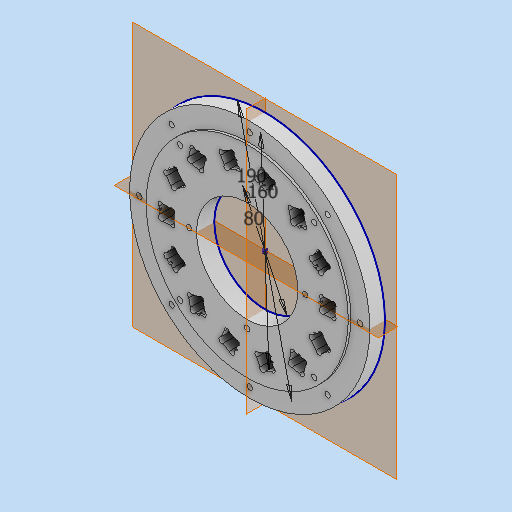
# Autodesk Inventor part: Ring 288_Final
Saved by Autodesk Inventor 2026 (Build 300175050, 175E)
## iProperties
Created: 2025-08-27
Part Number: Ring 288_Final
Material: Generic
Document SubType Name: Modeling
Designer: user
Density: 1 g/cm^3
Appearance: Default
Author: user
Autodesk Inventor part; units mm, degrees
sketch "Magnet Block n" plane through (0, 0, 0) normal (0, 0, 1) x (1, 0, 0)
  line L0 (69.7131, -5.94) -> (57.8331, -5.94)
  line L1 (57.8331, -5.94) -> (57.8331, 5.94)
  line L2 (57.8331, 5.94) -> (69.7131, 5.94)
  line L3 (69.7131, 5.94) -> (69.7131, -5.94)
  circle A0 centre (59.2461, 4.527) radius 2.1
  circle A1 centre (59.2461, -4.527) radius 2.1
  circle A2 centre (68.3001, -4.527) radius 2.1
  circle A3 centre (68.3001, 4.527) radius 2.1
  circle A4 centre (57.4731, 0) radius 0.75
  line L4 (57.4731, 0) -> (63.7731, 0)
  circle A5 centre (63.7731, 0) radius 2
  dimension "d10" = 4.2
  dimension "d11" = 4.2
  dimension "d12" = 4.2
  dimension "d13" = 4.2
  dimension "d8" = 11.88
  dimension "d9" = 11.88
  dimension "d18" = 1.5
  dimension "d19" = 6.3
  dimension "d20" = 4
  measures "d8" distance of point (57.833, 5.94) point (69.713, 5.94)
  measures "d9" distance of point (57.833, -5.94) point (57.833, 5.94)
  measures "d18" diameter of A4
  measures "d19" distance of L4.start L4.end
  measures "d20" diameter of A5
sketch "Sketch1" plane through (0, 0, 0) normal (0, 0, 1) x (1, 0, 0)
  circle A0 centre (0, 0) radius 40
  circle A1 centre (0, 0) radius 80
  circle A2 centre (0, 0) radius 95
  dimension "d0" = 80
  dimension "d1" = 160
  dimension "d2" = 190
  constraints: 3 centre point, 3 coincident
  measures "d0" diameter of A0
  measures "d1" diameter of A1
  measures "d2" diameter of A2
extrude "Extrusion1" add sketch "Sketch1" along normal blind 14 contours A1
extrude "Extrusion2" add sketch "Sketch1" along normal blind 12 contours A2
sketch "Sketch2" plane through (0, 0, 14) normal (0, 0, 1) x (1, 0, 0)
  circle A0 centre (0, 0) radius 63.7731
  line L0 (69.7131, -5.94) -> (57.8331, 5.94) construction
  line L1 (57.8331, -5.94) -> (69.7131, 5.94) construction
  line L2 (-112, 0) -> (112, 0) projected
  line L3 (69.7131, -5.94) -> (57.8331, -5.94)
  line L4 (57.8331, -5.94) -> (57.8331, 5.94)
  line L5 (57.8331, 5.94) -> (69.7131, 5.94)
  line L6 (69.7131, 5.94) -> (69.7131, -5.94)
  circle A1 centre (59.2461, 4.527) radius 2.1
  circle A2 centre (59.2461, -4.527) radius 2.1
  circle A3 centre (68.3001, -4.527) radius 2.1
  circle A4 centre (68.3001, 4.527) radius 2.1
  circle A5 centre (57.4731, 0) radius 0.75
  line L7 (57.4731, 0) -> (63.7731, 0)
  circle A6 centre (63.7731, 0) radius 2
  dimension "d7" = 127.5463
  constraints: 4 end point, 2 horizontal, 1 centre point, 1 coincident, 11 other
  measures "d7" diameter of A0
sketch "Sketch3" plane through (0, 0, 14) normal (0, 0, 1) x (1, 0, 0)
  circle A0 centre (0, 0) radius 63.7731
  line L0 (0, 0) -> (63.7731, 0)
  line L1 (0, 0) -> (57.4576, 27.6701)
  line L2 (0, 0) -> (39.7619, 49.8598)
  line L3 (0, 0) -> (14.1909, 62.1742)
  line L4 (0, 0) -> (-14.1909, 62.1742)
  line L5 (0, 0) -> (-39.7619, 49.8598)
  line L6 (0, 0) -> (-57.4576, 27.6701)
  line L7 (0, 0) -> (-63.7731, 0)
  line L8 (0, 0) -> (-57.4576, -27.6701)
  line L9 (0, 0) -> (-39.7619, -49.8598)
  line L10 (0, 0) -> (-14.1909, -62.1742)
  line L11 (0, 0) -> (14.1909, -62.1742)
  line L12 (0, 0) -> (39.7619, -49.8598)
  line L13 (0, 0) -> (57.4576, -27.6701)
  line L14 (69.7131, -5.94) -> (57.8331, -5.94)
  line L15 (57.8331, -5.94) -> (57.8331, 5.94)
  line L16 (57.8331, 5.94) -> (69.7131, 5.94)
  line L17 (69.7131, 5.94) -> (69.7131, -5.94)
  circle A1 centre (59.2461, 4.527) radius 2.1
  circle A2 centre (59.2461, -4.527) radius 2.1
  circle A3 centre (68.3001, -4.527) radius 2.1
  circle A4 centre (68.3001, 4.527) radius 2.1
  circle A5 centre (57.4731, 0) radius 0.75
  line L18 (57.4731, 0) -> (63.7731, 0)
  circle A6 centre (63.7731, 0) radius 2
  line L19 (65.8052, 28.6107) -> (58.3982, 19.3225)
  line L20 (58.3982, 19.3225) -> (49.11, 26.7296)
  line L21 (49.11, 26.7296) -> (56.5171, 36.0177)
  line L22 (56.5171, 36.0177) -> (65.8052, 28.6107)
  circle A7 centre (51.0957, 26.9533) radius 2.1
  circle A8 centre (58.1744, 21.3082) radius 2.1
  circle A9 centre (63.8195, 28.3869) radius 2.1
  circle A10 centre (56.7408, 34.032) radius 2.1
  circle A11 centre (53.5296, 22.7446) radius 0.75
  line L23 (53.5296, 22.7446) -> (57.4576, 27.6701)
  circle A12 centre (57.4576, 27.6701) radius 2
  line L24 (44.2312, 56.9727) -> (46.8747, 45.3906)
  line L25 (46.8747, 45.3906) -> (35.2926, 42.747)
  line L26 (35.2926, 42.747) -> (32.6491, 54.3291)
  line L27 (32.6491, 54.3291) -> (44.2312, 56.9727)
  circle A13 centre (36.3558, 44.439) radius 2.1
  circle A14 centre (45.1828, 46.4537) radius 2.1
  circle A15 centre (43.168, 55.2807) radius 2.1
  circle A16 centre (34.3411, 53.266) radius 2.1
  circle A17 centre (41.1638, 43.7178) radius 0.75
  line L28 (41.1638, 43.7178) -> (39.7619, 49.8598)
  circle A18 centre (39.7619, 49.8598) radius 2
  line L29 (11.4164, 70.1032) -> (22.1199, 64.9487)
  line L30 (22.1199, 64.9487) -> (16.9653, 54.2452)
  line L31 (16.9653, 54.2452) -> (6.2618, 59.3997)
  line L32 (6.2618, 59.3997) -> (11.4164, 70.1032)
  circle A19 centre (16.3054, 56.1313) radius 2.1
  circle A20 centre (20.2337, 64.2887) radius 2.1
  circle A21 centre (12.0764, 68.2171) radius 2.1
  circle A22 centre (8.148, 60.0597) radius 2.1
  circle A23 centre (19.867, 59.4407) radius 0.75
  line L33 (19.867, 59.4407) -> (14.1909, 62.1742)
  circle A24 centre (14.1909, 62.1742) radius 2
  line L34 (-22.1199, 64.9487) -> (-11.4164, 70.1032)
  line L35 (-11.4164, 70.1032) -> (-6.2618, 59.3997)
  line L36 (-6.2618, 59.3997) -> (-16.9653, 54.2452)
  line L37 (-16.9653, 54.2452) -> (-22.1199, 64.9487)
  circle A25 centre (-8.148, 60.0597) radius 2.1
  circle A26 centre (-12.0764, 68.2171) radius 2.1
  circle A27 centre (-20.2337, 64.2887) radius 2.1
  circle A28 centre (-16.3054, 56.1313) radius 2.1
  circle A29 centre (-8.5148, 64.9077) radius 0.75
  line L38 (-8.5148, 64.9077) -> (-14.1909, 62.1742)
  circle A30 centre (-14.1909, 62.1742) radius 2
  line L39 (-46.8747, 45.3906) -> (-44.2312, 56.9727)
  line L40 (-44.2312, 56.9727) -> (-32.6491, 54.3291)
  line L41 (-32.6491, 54.3291) -> (-35.2926, 42.747)
  line L42 (-35.2926, 42.747) -> (-46.8747, 45.3906)
  circle A31 centre (-34.3411, 53.266) radius 2.1
  circle A32 centre (-43.168, 55.2807) radius 2.1
  circle A33 centre (-45.1828, 46.4537) radius 2.1
  circle A34 centre (-36.3558, 44.439) radius 2.1
  circle A35 centre (-38.36, 56.0019) radius 0.75
  line L43 (-38.36, 56.0019) -> (-39.7619, 49.8598)
  circle A36 centre (-39.7619, 49.8598) radius 2
  line L44 (-58.3982, 19.3225) -> (-65.8052, 28.6107)
  line L45 (-65.8052, 28.6107) -> (-56.5171, 36.0177)
  line L46 (-56.5171, 36.0177) -> (-49.11, 26.7296)
  line L47 (-49.11, 26.7296) -> (-58.3982, 19.3225)
  circle A37 centre (-56.7408, 34.032) radius 2.1
  circle A38 centre (-63.8195, 28.3869) radius 2.1
  circle A39 centre (-58.1744, 21.3082) radius 2.1
  circle A40 centre (-51.0957, 26.9533) radius 2.1
  circle A41 centre (-61.3856, 32.5957) radius 0.75
  line L48 (-61.3856, 32.5957) -> (-57.4576, 27.6701)
  circle A42 centre (-57.4576, 27.6701) radius 2
  line L49 (-57.8331, -5.94) -> (-69.7131, -5.94)
  line L50 (-69.7131, -5.94) -> (-69.7131, 5.94)
  line L51 (-69.7131, 5.94) -> (-57.8331, 5.94)
  line L52 (-57.8331, 5.94) -> (-57.8331, -5.94)
  circle A43 centre (-68.3001, 4.527) radius 2.1
  circle A44 centre (-68.3001, -4.527) radius 2.1
  circle A45 centre (-59.2461, -4.527) radius 2.1
  circle A46 centre (-59.2461, 4.527) radius 2.1
  circle A47 centre (-70.0731, 0) radius 0.75
  line L53 (-70.0731, 0) -> (-63.7731, 0)
  circle A48 centre (-63.7731, 0) radius 2
  line L54 (-49.11, -26.7296) -> (-56.5171, -36.0177)
  line L55 (-56.5171, -36.0177) -> (-65.8052, -28.6107)
  line L56 (-65.8052, -28.6107) -> (-58.3982, -19.3225)
  line L57 (-58.3982, -19.3225) -> (-49.11, -26.7296)
  circle A49 centre (-63.8195, -28.3869) radius 2.1
  circle A50 centre (-56.7408, -34.032) radius 2.1
  circle A51 centre (-51.0957, -26.9533) radius 2.1
  circle A52 centre (-58.1744, -21.3082) radius 2.1
  circle A53 centre (-61.3856, -32.5957) radius 0.75
  line L58 (-61.3856, -32.5957) -> (-57.4576, -27.6701)
  circle A54 centre (-57.4576, -27.6701) radius 2
  line L59 (-35.2926, -42.747) -> (-32.6491, -54.3291)
  line L60 (-32.6491, -54.3291) -> (-44.2312, -56.9727)
  line L61 (-44.2312, -56.9727) -> (-46.8747, -45.3906)
  line L62 (-46.8747, -45.3906) -> (-35.2926, -42.747)
  circle A55 centre (-43.168, -55.2807) radius 2.1
  circle A56 centre (-34.3411, -53.266) radius 2.1
  circle A57 centre (-36.3558, -44.439) radius 2.1
  circle A58 centre (-45.1828, -46.4537) radius 2.1
  circle A59 centre (-38.36, -56.0019) radius 0.75
  line L63 (-38.36, -56.0019) -> (-39.7619, -49.8598)
  circle A60 centre (-39.7619, -49.8598) radius 2
  line L64 (-16.9653, -54.2452) -> (-6.2618, -59.3997)
  line L65 (-6.2618, -59.3997) -> (-11.4164, -70.1032)
  line L66 (-11.4164, -70.1032) -> (-22.1199, -64.9487)
  line L67 (-22.1199, -64.9487) -> (-16.9653, -54.2452)
  circle A61 centre (-12.0764, -68.2171) radius 2.1
  circle A62 centre (-8.148, -60.0597) radius 2.1
  circle A63 centre (-16.3054, -56.1313) radius 2.1
  circle A64 centre (-20.2337, -64.2887) radius 2.1
  circle A65 centre (-8.5148, -64.9077) radius 0.75
  line L68 (-8.5148, -64.9077) -> (-14.1909, -62.1742)
  circle A66 centre (-14.1909, -62.1742) radius 2
  line L69 (6.2618, -59.3997) -> (16.9653, -54.2452)
  line L70 (16.9653, -54.2452) -> (22.1199, -64.9487)
  line L71 (22.1199, -64.9487) -> (11.4164, -70.1032)
  line L72 (11.4164, -70.1032) -> (6.2618, -59.3997)
  circle A67 centre (20.2337, -64.2887) radius 2.1
  circle A68 centre (16.3054, -56.1313) radius 2.1
  circle A69 centre (8.148, -60.0597) radius 2.1
  circle A70 centre (12.0764, -68.2171) radius 2.1
  circle A71 centre (19.867, -59.4407) radius 0.75
  line L73 (19.867, -59.4407) -> (14.1909, -62.1742)
  circle A72 centre (14.1909, -62.1742) radius 2
  line L74 (32.6491, -54.3291) -> (35.2926, -42.747)
  line L75 (35.2926, -42.747) -> (46.8747, -45.3906)
  line L76 (46.8747, -45.3906) -> (44.2312, -56.9727)
  line L77 (44.2312, -56.9727) -> (32.6491, -54.3291)
  circle A73 centre (45.1828, -46.4537) radius 2.1
  circle A74 centre (36.3558, -44.439) radius 2.1
  circle A75 centre (34.3411, -53.266) radius 2.1
  circle A76 centre (43.168, -55.2807) radius 2.1
  circle A77 centre (41.1638, -43.7178) radius 0.75
  line L78 (41.1638, -43.7178) -> (39.7619, -49.8598)
  circle A78 centre (39.7619, -49.8598) radius 2
  line L79 (56.5171, -36.0177) -> (49.11, -26.7296)
  line L80 (49.11, -26.7296) -> (58.3982, -19.3225)
  line L81 (58.3982, -19.3225) -> (65.8052, -28.6107)
  line L82 (65.8052, -28.6107) -> (56.5171, -36.0177)
  circle A79 centre (58.1744, -21.3082) radius 2.1
  circle A80 centre (51.0957, -26.9533) radius 2.1
  circle A81 centre (56.7408, -34.032) radius 2.1
  circle A82 centre (63.8195, -28.3869) radius 2.1
  circle A83 centre (53.5296, -22.7446) radius 0.75
  line L83 (53.5296, -22.7446) -> (57.4576, -27.6701)
  circle A84 centre (57.4576, -27.6701) radius 2
  point P0 (-8.9346, 58.1126)
  point P1 (-7.549, 62.0725)
  point P2 (-10.1292, 67.4305)
  point P3 (-14.0891, 68.8161)
  point P4 (-19.4471, 66.2358)
  point P5 (-20.8328, 62.276)
  point P6 (-18.2525, 56.9179)
  point P7 (-14.2926, 55.5323)
  point P8 (-41.3391, 56.3126)
  point P9 (-44.8913, 54.0805)
  point P10 (-46.2146, 48.2827)
  point P11 (-43.9826, 44.7304)
  point P12 (-38.1848, 43.4071)
  point P13 (-34.6325, 45.6391)
  point P14 (-33.3092, 51.437)
  point P15 (-35.5412, 54.9893)
  point P16 (-54.6675, 33.6984)
  point P17 (-58.8364, 34.1681)
  point P18 (-63.4859, 30.4603)
  point P19 (-63.9556, 26.2914)
  point P20 (-60.2478, 21.6418)
  point P21 (-56.0788, 21.1721)
  point P22 (-51.4293, 24.88)
  point P23 (-50.9596, 29.0489)
  point P24 (-69.7131, -2.9735)
  point P25 (-66.7466, -5.94)
  point P26 (-60.7997, -5.94)
  point P27 (-57.8331, -2.9735)
  point P28 (-57.8331, 2.9735)
  point P29 (-60.7997, 5.94)
  point P30 (-66.7466, 5.94)
  point P31 (-69.7131, 2.9735)
  point P32 (-56.0788, -21.1721)
  point P33 (-60.2478, -21.6418)
  point P34 (-63.9556, -26.2914)
  point P35 (-63.4859, -30.4603)
  point P36 (-58.8364, -34.1681)
  point P37 (-54.6675, -33.6984)
  point P38 (-50.9596, -29.0489)
  point P39 (-51.4293, -24.88)
  point P40 (-33.3092, -51.437)
  point P41 (-34.6325, -45.6391)
  point P42 (-38.1848, -43.4071)
  point P43 (-43.9826, -44.7304)
  point P44 (-46.2146, -48.2827)
  point P45 (-44.8913, -54.0805)
  point P46 (-41.3391, -56.3126)
  point P47 (-35.5412, -54.9893)
  point P48 (-20.8328, -62.276)
  point P49 (-19.4471, -66.2358)
  point P50 (-14.0891, -68.8161)
  point P51 (-10.1292, -67.4305)
  point P52 (-7.549, -62.0725)
  point P53 (-8.9346, -58.1126)
  point P54 (-14.2926, -55.5323)
  point P55 (-18.2525, -56.9179)
  point P56 (18.2525, -56.9179)
  point P57 (14.2926, -55.5323)
  point P58 (8.9346, -58.1126)
  point P59 (7.549, -62.0725)
  point P60 (10.1292, -67.4305)
  point P61 (14.0891, -68.8161)
  point P62 (19.4471, -66.2358)
  point P63 (20.8328, -62.276)
  point P64 (38.1848, -43.4071)
  point P65 (34.6325, -45.6391)
  point P66 (33.3092, -51.437)
  point P67 (35.5412, -54.9893)
  point P68 (41.3391, -56.3126)
  point P69 (44.8913, -54.0805)
  point P70 (46.2146, -48.2827)
  point P71 (43.9826, -44.7304)
  point P72 (63.4859, -30.4603)
  point P73 (63.9556, -26.2914)
  point P74 (60.2478, -21.6418)
  point P75 (56.0788, -21.1721)
  point P76 (51.4293, -24.88)
  point P77 (50.9596, -29.0489)
  point P78 (54.6675, -33.6984)
  point P79 (58.8364, -34.1681)
  point P80 (57.8331, -2.9735)
  point P81 (60.7997, -5.94)
  point P82 (66.7466, -5.94)
  point P83 (69.7131, -2.9735)
  point P84 (69.7131, 2.9735)
  point P85 (66.7466, 5.94)
  point P86 (60.7997, 5.94)
  point P87 (57.8331, 2.9735)
  point P88 (56.0788, 21.1721)
  point P89 (60.2403, 20.9313)
  point P90 (60.0691, 21.4178)
  point P91 (63.9556, 26.2914)
  point P92 (63.4859, 30.4603)
  point P93 (58.8364, 34.1681)
  point P94 (54.6675, 33.6984)
  point P95 (50.9596, 29.0489)
  point P96 (51.4293, 24.88)
  point P97 (14.2926, 55.5323)
  point P98 (18.2525, 56.9179)
  point P99 (20.8328, 62.276)
  point P100 (19.4471, 66.2358)
  point P101 (14.0891, 68.8161)
  point P102 (10.1292, 67.4305)
  point P103 (7.549, 62.0725)
  point P104 (8.9346, 58.1126)
  point P105 (33.3092, 51.437)
  point P106 (34.6325, 45.6391)
  point P107 (38.1848, 43.4071)
  point P108 (43.9826, 44.7304)
  point P109 (46.2146, 48.2827)
  point P110 (44.8913, 54.0805)
  point P111 (41.3391, 56.3126)
  point P112 (35.5412, 54.9893)
  point P113 (-37.7987, 55.5045)
  point P114 (-39.0816, 55.7973)
  dimension "d21" = 127.5463
  dimension "d24" = 360
  dimension "d26" = 0
  dimension "d27" = -51.429
  dimension "d28" = -102.857
  dimension "d29" = -154.286
  dimension "d30" = -205.714
  dimension "d31" = -257.143
  dimension "d33" = 180
  dimension "d34" = -51.429
  dimension "d35" = -102.857
  dimension "d36" = -154.286
  dimension "d37" = -205.714
  dimension "d38" = 77.143
  dimension "d39" = 128.571
  dimension "d46" = 128.571
  constraints: 28 end point, 1 coincident, 1 horizontal, 60 other
  measures "d26" vertical extent of L0
  measures "d33" angle to the sketch x axis of L0
extrude "Extrusion3" cut sketch "Sketch3" against normal blind 12 contours L0 A6 A0 | A0 A6 | A0 A6 L0 | A6 L0 A5 L15 A1 L16 A0 | A0 L16 A4 L17 A3 L14 A6 | A0 L14 A2 L15 A5 L0 A6 | A5 L15 L0 | L0 L15 A5 | A8 L20 L19 A0 | A1 L15 L16 | L16 L15 A1 | A4 L17 L16 | L16 L17 A4 | A79 L81 A0 | A0 L81 L80 A79 | A3 L17 L14 | L14 L17 A3 | A2 L15 L14 | L14 L15 A2 | L19 L20 A8 A0 | A0 A8 L19 | L20 A11 L23 A12 A0 A8 | L81 A79 A0 | A0 A79 L80 L81 | A79 A0 A84 L83 A83 L80 | A0 A12 L21 A10 L22 A9 L19 A8 | L20 L23 A11 | A79 L81 A82 L82 A81 L79 A0 A84 | A83 L83 L80 | A12 L23 A0 | A0 A12 | A9 L22 L19 | L19 L22 A9 | L20 A11 L23 | L20 L1 A12 L23 A11 | A84 A0 | A0 L83 A84 | A82 L82 L81 | L81 L82 A82 | L83 A83 L80 | A83 L83 A84 L13 L80 | L20 A7 L21 A0 A12 L1 | A13 L26 L2 | L2 L26 L25 A13 | L31 A22 L32 A0 A24 L3 | L3 A24 L33 A23 L30 A19 L31 | L36 A28 L37 A0 A30 L4 | L4 A30 A0 L35 A25 L36 | A34 L42 L41 L5 | L5 L41 A34 | L47 A39 A0 A42 L6 | L6 A42 A0 L46 A40 L47 | L52 A45 L49 A0 A48 L7 | L7 A48 A0 L51 A46 L52 | L57 A51 L54 A0 A54 L8 | L8 A54 A0 A52 L57 | A57 L59 L9 | L9 L59 L62 A57 | L64 A62 L65 A0 A66 L10 | L10 A66 A0 L67 A63 L64 | L69 A68 L70 A71 L73 A72 L11 | L11 A72 A0 L72 A69 L69 | A74 L75 L74 L12 | L12 L74 A74 | L13 A84 A0 L79 A80 L80 | L1 A12 A0 | L23 A12 L1 | A0 A84 L13 | L13 A84 L83 | A7 L21 L20 | L20 L21 A7 | L26 A13 L2 | L2 A13 L25 L26 | L26 A16 A0 A18 L2 A13 | A13 L2 A18 L28 A17 L25 | A24 A0 L3 | L3 L33 A24 | A19 L30 L31 | L31 L30 A19 | A22 L32 L31 | L31 L32 A22 | A30 A0 L4 | L4 A0 A30 | A25 L35 L36 | L36 L35 A25 | A28 L37 L36 | L36 L37 A28 | L41 L42 A34 L5 | L5 A34 L41 | L42 A33 A0 A36 L5 A34 | A42 A0 L6 | L6 A0 A42 | A40 L46 L47 | L47 L46 A40 | A39 A0 L44 L47 | L47 L44 A0 A39 | A48 A0 L7 | L7 A0 A48 | A46 L51 L52 | L52 L51 A46 | A45 L49 L52 | L52 L49 A45 | A54 A0 L8 | L8 A0 A54 | A52 A0 L56 L57 | L57 L56 A0 A52 | A51 L54 L57 | L57 L54 A51 | L59 A57 L9 | L9 A57 L62 L59 | A57 L9 A60 A0 A58 L62 | A66 A0 L10 | L10 A0 A66 | A63 L67 L64 | L64 L67 A63 | A62 L65 L64 | L64 L65 A62 | A72 L73 L11 | L11 A0 A72 | A69 L72 L69 | L69 L72 A69 | A68 L70 L69 | L69 L70 A68 | L74 L75 A74 L12 | L12 A74 L74 | L75 A77 L78 A78 L12 A74 | A74 L12 A78 A0 A75 L74 | A80 L79 L80 | L80 L79 A80 | A10 L21 L22 | L22 L21 A10 | A81 L79 L82 | L82 L79 A81 | A16 A0 L27 L26 | L26 L27 A0 A16 | A17 L28 L25 | A0 A24 | A0 A24 L33 | A0 L32 A21 L29 A20 L30 A24 | A24 A0 L30 A23 L33 | L38 A30 A0 | A0 A30 L38 | A0 L37 A27 L34 A26 L35 A29 L38 A30 | L5 A36 A0 A31 L41 A34 | A33 A0 L42 | L42 A0 A33 | L48 A42 A0 | A0 A42 L48 | A0 A39 L44 A38 L45 A41 L48 A42 | A39 L44 A0 | L53 A48 A0 | A0 A48 L53 | A48 L53 A47 L50 A43 L51 A0 | A0 L49 A44 L50 A47 L53 A48 | L58 A54 A0 | A0 A54 L58 | A54 L58 A53 L55 A49 L56 A52 A0 | A0 L56 A52 | A57 L59 A56 A0 A60 L9 | A58 A0 L62 | L62 A0 A58 | L68 A66 A0 | A0 A66 L68 | A66 L68 A65 L65 A61 L66 A64 L67 A0 | A0 A72 | L73 A72 A0 | L73 A71 L70 A0 A72 | A72 A0 L70 A67 L71 A70 L72 | L75 L78 A77 | A75 A0 L77 L74 | L74 L77 A0 A75 | A18 A0 L2 | L2 L28 A18 | A16 L27 A0 | A16 L27 A15 L24 A14 A0 A18 | A0 L27 A16 | L28 A17 L25 | L28 A18 A0 A14 L25 A17 | L33 L30 A23 | A23 L30 L33 | A30 L38 A29 L35 A0 | A36 A0 L5 | L5 A0 A36 | A31 A0 L40 L41 | L41 L40 A0 A31 | L42 L39 A33 A0 | A0 A33 L39 L42 | A42 L48 A41 L45 A37 L46 A0 | A0 L44 A39 | A0 L54 A50 L55 A53 L58 A54 | A52 L56 A0 | A60 A0 L9 | L9 A0 A60 | A56 A0 L60 L59 | L59 L60 A0 A56 | L62 L61 A58 A0 | A0 A58 L61 L62 | A0 L65 A65 L68 A66 | L73 L70 A71 | A71 L70 L73 | A78 L78 L12 | L12 A0 A78 | L75 A77 L78 | A77 L75 A73 A0 A78 L78 | A75 L77 A0 | A0 A78 A73 L76 A76 L77 A75 | A0 L77 A75 | A14 L25 A0 | A0 L25 L24 A14 | A73 L76 L75 A0 | A0 L75 A73 | A0 A18 | A0 A18 L28 | A21 L29 L32 | L32 L29 A21 | L38 L35 A29 | A29 L35 L38 | A0 L40 A31 | A27 L34 L37 | L37 L34 A27 | L43 A36 A0 | A0 A36 L43 | A0 A33 L39 A32 L40 A35 L43 A36 | A31 L40 A0 | A0 A36 L43 A35 L40 A31 | L48 L45 A41 | A41 L45 L48 | A37 L45 L46 | L46 L45 A37 | A43 L50 L51 | L51 L50 A43 | A38 L45 L44 | L44 L45 A38 | L53 L50 A47 | A47 L50 L53 | A44 L50 L49 | L49 L50 A44 | L58 L55 A53 | A53 L55 L58 | A49 L55 L56 | L56 L55 A49 | A50 L55 L54 | L54 L55 A50 | L63 A60 A0 | A0 A60 L63 | A60 L63 A59 L60 A55 L61 A58 A0 | A56 L60 A59 L63 A60 A0 | A0 L60 A56 | L68 L65 A65 | A65 L65 L68 | A56 L60 A0 | A64 L66 L67 | L67 L66 A64 | A70 L71 L72 | L72 L71 A70 | A0 A78 | L78 A78 A0 | L25 A14 A0 | A0 A14 L24 L25 | L75 L76 A73 A0 | A0 A73 L75 | A20 L29 L30 | L30 L29 A20 | A15 L24 L27 | L27 L24 A15 | A32 L40 L39 | L39 L40 A32 | A55 L60 L61 | L61 L60 A55 | A67 L71 L70 | L70 L71 A67 | A76 L76 L77 | L77 L76 A76 | A26 L34 L35 | L35 L34 A26 | A35 L43 L40 | A35 L40 L43 | L63 L60 A59 | A59 L60 L63 | A61 L66 L65 | L65 L66 A61 picked at (57.8769, -0.4081) picked at (57.8769, 0.4081) picked at (59.8979, 22.1594)
extrude "Extrusion4" cut sketch "Sketch3" against normal blind 2 contours A5 L15 L0 | L0 L15 A5 | L15 A5 L0 | L0 A5 L15 | A11 L20 | L20 L23 A11 | A83 L83 L80 | L80 A83 | L20 A11 L23 | L83 A83 L80 | A17 L28 L25 | L25 A17 | A77 L75 | L75 L78 A77 | L28 A17 L25 | L33 L30 A23 | A23 L30 L33 | L30 A23 | L73 L70 A71 | A71 L70 L73 | A71 L70 | L75 A77 L78 | L38 L35 A29 | A29 L35 L38 | L35 A29 | L48 L45 A41 | A41 L45 L48 | L53 L50 A47 | A47 L50 L53 | L58 L55 A53 | A53 L55 L58 | L68 L65 A65 | A65 L65 L68 | A65 L65 | A41 L45 | L50 A47 | L55 A53 | L40 A35 | L63 L60 A59 | A59 L60 L63 | A59 L60
extrude "Extrusion5" cut sketch "Sketch3" against normal through all contours L0 A6 A0 | A0 A6 | A0 A6 L0 | A12 L23 A0 | A0 A12 | A84 A0 | A0 L83 A84 | L1 A12 A0 | L23 A12 L1 | A0 A84 L13 | L13 A84 L83 | A24 A0 L3 | L3 L33 A24 | A30 A0 L4 | L4 A0 A30 | A42 A0 L6 | L6 A0 A42 | A48 A0 L7 | L7 A0 A48 | A54 A0 L8 | L8 A0 A54 | A66 A0 L10 | L10 A0 A66 | A72 L73 L11 | L11 A0 A72 | A0 A24 | A0 A24 L33 | L38 A30 A0 | A0 A30 L38 | L48 A42 A0 | A0 A42 L48 | L53 A48 A0 | A0 A48 L53 | L58 A54 A0 | A0 A54 L58 | L68 A66 A0 | A0 A66 L68 | A0 A72 | L73 A72 A0 | A18 A0 L2 | L2 L28 A18 | A36 A0 L5 | L5 A0 A36 | A60 A0 L9 | L9 A0 A60 | A78 L78 L12 | L12 A0 A78 | A0 A18 | A0 A18 L28 | L43 A36 A0 | A0 A36 L43 | L63 A60 A0 | A0 A60 L63 | A0 A78 | L78 A78 A0
sketch "Sketch4" plane through (0, 0, 14) normal (0, 0, 1) x (1, 0, 0)
  circle A0 centre (46, 0) radius 2.1
  circle A1 centre (0, 46) radius 2.1
  circle A2 centre (-46, 0) radius 2.1
  circle A3 centre (0, -46) radius 2.1
  point P0 (0, 0)
  dimension "d47" = 4.2
  dimension "d50" = 360
  dimension "d52" = 46
  constraints: 4 centre point, 9 other
  measures "d47" diameter of A0
  measures "d52" distance of A0.centre point (0, 0)
extrude "Extrusion6" cut sketch "Sketch4" against normal blind 10
sketch "Sketch5" plane through (0, 0, 12) normal (0, 0, 1) x (1, 0, 0)
  circle A0 centre (87.25, 0) radius 2.15
  circle A1 centre (61.6951, 61.6951) radius 2.15
  circle A2 centre (0, 87.25) radius 2.15
  circle A3 centre (-61.6951, 61.6951) radius 2.15
  circle A4 centre (-87.25, 0) radius 2.15
  circle A5 centre (-61.6951, -61.6951) radius 2.15
  circle A6 centre (0, -87.25) radius 2.15
  circle A7 centre (61.6951, -61.6951) radius 2.15
  point P0 (0, 0)
  dimension "d55" = 4.3
  dimension "d56" = 87.25
  dimension "d59" = 360
  constraints: 8 centre point, 17 other
  measures "d55" diameter of A0
  measures "d56" distance of A0.centre point (0, 0)
extrude "Extrusion7" cut sketch "Sketch5" against normal blind 14
sketch "Sketch6" plane through (0, 0, 14) normal (0, 0, 1) x (1, 0, 0)
  circle A0 centre (0, 0) radius 75
  circle A1 centre (53.033, 53.033) radius 2.1
  line L0 (53.033, 53.033) -> (0, 0)
  line L1 (-133, 0) -> (133, 0) projected
  circle A2 centre (-53.033, 53.033) radius 2.1
  circle A3 centre (-53.033, -53.033) radius 2.1
  circle A4 centre (53.033, -53.033) radius 2.1
  dimension "d63" = 150
  dimension "d64" = 4.2
  dimension "d65" = 45
  dimension "d68" = 360
  constraints: 4 centre point, 3 coincident, 2 end point, 14 other
  measures "d64" diameter of A1
  measures "d65" angle of L1 L0
extrude "Extrusion8" cut sketch "Sketch6" against normal blind 10 contours A1 L0 A0 | A0 A1 | A4 A0 | A0 A4 | L0 A1 A0 | A3 A0 | A0 A3 | A2 A0 | A0 A2
body "Solid1"
